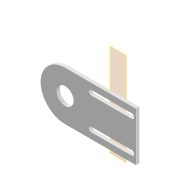
# Autodesk Inventor part: driven wheel arm
Saved by Autodesk Inventor 2020 (Build 240168000, 168)
## iProperties
Created: 2020-01-25
Part Number: driven wheel arm
Material: Generic
Document SubType Name: Modeling
Designer: ball
Density: 1 g/cm^3
Appearance: Default
Author: ball
Autodesk Inventor part; units mm, degrees
ref_plane "YZ Plane" through (0, 0, 0) normal (1, 0, 0) x (0, 1, 0)
ref_plane "XZ Plane" through (0, 0, 0) normal (0, 1, 0) x (-1, 0, 0)
ref_plane "XY Plane" through (0, 0, 0) normal (0, 0, 1) x (1, 0, 0)
ref_plane "Work Plane1" through (0, 0, 0) normal (0, 0, 1) x (1, 0, 0)
sketch "Sketch1" plane through (0, 0, 0) normal (0, 0, 1) x (1, 0, 0)
  line L0 (11.43, 0) -> (11.43, -63.5) construction
  line L1 (0, 0) -> (11.43, 0) construction
  line L2 (0, 0) -> (0, -63.5) construction
  line L3 (7.44, -34.7378) -> (0, -34.7378) construction
  circle A0 centre (5.715, -31.75) radius 1.7 construction
  circle A1 centre (-31.5722, -43.7048) radius 6.4135
  line L4 (0, -63.5) -> (11.43, -63.5) construction
  circle A2 centre (5.715, -55.6597) radius 1.7 construction
  line L5 (21.59, -62.0097) -> (-31.5722, -62.0097)
  line L6 (-31.5722, -25.4) -> (21.59, -25.4)
  line L7 (21.59, -25.4) -> (21.59, -62.0097)
  arc A3 (-31.5722, -25.4) -> (-31.5722, -62.0097) centre (-31.5722, -43.7048) ccw
  line L8 (18.415, -31.75) -> (-12.065, -31.75) construction
  line L9 (18.415, -29.95) -> (-12.065, -29.95)
  line L10 (-12.065, -33.55) -> (18.415, -33.55)
  arc A4 (18.415, -33.55) -> (18.415, -29.95) centre (18.415, -31.75) ccw
  arc A5 (-12.065, -29.95) -> (-12.065, -33.55) centre (-12.065, -31.75) ccw
  line L11 (18.415, -55.6597) -> (-12.065, -55.6597) construction
  line L12 (18.415, -53.8597) -> (-12.065, -53.8597)
  line L13 (-12.065, -57.4597) -> (18.415, -57.4597)
  arc A6 (18.415, -57.4597) -> (18.415, -53.8597) centre (18.415, -55.6597) ccw
  arc A7 (-12.065, -53.8597) -> (-12.065, -57.4597) centre (-12.065, -55.6597) ccw
  point P0 (3.175, -31.75)
  point P1 (3.175, -55.6597)
extrude "Extrusion1" add sketch "Sketch1" along normal blind 2.5
equation "\"d3\" = d4 + 0.5 * d5"
equation "\"d4\" = 7.8403"
equation "\"d5\" = 23.9097"
body "Solid1"
